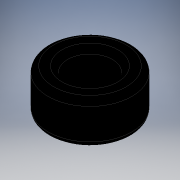
# Autodesk Inventor part: coil
Saved by Autodesk Inventor 2019 (Build 230136000, 136)
## iProperties
Created: 2022-02-03
Part Number: coil
Material: Generic
Document SubType Name: Modeling
Designer: josec
Density: 1 g/cm^3
Appearance: Default
Author: josec
Autodesk Inventor part; units mm, degrees
ref_plane "YZ Plane" through (0, 0, 0) normal (1, 0, 0) x (0, 1, 0)
ref_plane "XZ Plane" through (0, 0, 0) normal (0, 1, 0) x (-1, 0, 0)
ref_plane "XY Plane" through (0, 0, 0) normal (0, 0, 1) x (1, 0, 0)
sketch "Sketch1" plane through (0, 0, 0) normal (0, 1, 0) x (-1, 0, 0)
  point P0 (0, 0)
sketch "Sketch2" plane through (0, 0, 0) normal (0, 1, 0) x (-1, 0, 0)
  circle A0 centre (0, 0) radius 8
  circle A1 centre (0, 0) radius 15
  dimension "d0" = 16
  dimension "d1" = 30
  constraints: 2 centre point, 2 coincident
  measures "d0" diameter of A0
  measures "d1" diameter of A1
extrude "Extrusion1" add sketch "Sketch2" along normal blind 15
fillet "Fillet1" radius 2 1 edges at (15, 15, 0)
fillet "Fillet2" radius 2 1 edges at (8, 15, 0)
fillet "Fillet3" radius 2 2 edges at (15, 0, 0) (8, 0, 0)
body "Solid1"
